Autodesk Inventor part; units mm, degrees
(part 2 of 2)
  spline S373 degree 2 poles (72.0686, 10.5759) (71.9893, 11.231) (71.9893, 11.5552) knots 0 0 0 1 1 1
  spline S374 degree 2 poles (76.8272, 9.9966) (76.7652, 9.9966) (76.541, 10.0724) (76.479, 10.0724) knots 0 0 0 1 2 2 2
  spline S375 degree 2 poles (76.479, 10.0724) (76.3548, 10.0724) (75.8514, 10.0414) (75.7203, 10.0414) knots 0 0 0 1 2 2 2
  spline S376 degree 2 poles (75.7203, 10.0414) (75.6238, 10.0414) (75.2479, 9.9931) (75.1514, 9.9931) knots 0 0 0 1 2 2 2
  spline S377 degree 2 poles (75.1514, 9.9931) (75.1238, 9.9931) (75.0203, 10.0138) (74.9927, 10.0138) knots 0 0 0 1 2 2 2
  spline S378 degree 2 poles (74.9927, 10.0138) (74.8238, 10.0138) (74.7721, 10.1793) knots 0 0 0 1 1 1
  spline S379 degree 2 poles (74.7721, 10.1793) (74.741, 10.2655) (74.741, 10.4759) knots 0 0 0 1 1 1
  spline S380 degree 2 poles (74.741, 10.4759) (74.741, 11.0517) (75.0548, 11.4034) knots 0 0 0 1 1 1
  spline S381 degree 2 poles (75.0548, 11.4034) (75.1996, 11.5621) (75.8272, 11.9966) knots 0 0 0 1 1 1
  spline S382 degree 2 poles (75.8272, 11.9966) (76.1824, 12.2379) (76.2996, 12.3759) knots 0 0 0 1 1 1
  spline S383 degree 2 poles (76.2996, 12.3759) (76.5134, 12.6103) (76.5134, 12.931) knots 0 0 0 1 1 1
  spline S384 degree 2 poles (76.5134, 12.931) (76.5134, 13.0897) (76.31, 13.2138) knots 0 0 0 1 1 1
  spline S385 degree 2 poles (76.31, 13.2138) (76.1272, 13.3241) (75.9548, 13.3241) knots 0 0 0 1 1 1
  spline S386 degree 2 poles (75.9548, 13.3241) (75.7272, 13.3241) (75.5238, 13.1931) knots 0 0 0 1 1 1
  line L70 (75.5238, 13.1931) -> (75.1686, 12.9138)
  spline S387 degree 2 poles (75.1686, 12.9138) (75.0617, 12.831) (74.9996, 12.831) knots 0 0 0 1 1 1
  spline S388 degree 2 poles (74.9996, 12.831) (74.7445, 12.831) (74.7445, 13.0345) knots 0 0 0 1 1 1
  spline S389 degree 2 poles (74.7445, 13.0345) (74.7445, 13.1517) (74.8376, 13.2345) knots 0 0 0 1 1 1
  spline S390 degree 2 poles (74.8376, 13.2345) (75.1272, 13.5069) (75.341, 13.6276) knots 0 0 0 1 1 1
  spline S391 degree 2 poles (75.341, 13.6276) (75.6376, 13.8) (75.9548, 13.8) knots 0 0 0 1 1 1
  spline S392 degree 2 poles (75.9548, 13.8) (76.3548, 13.8) (76.6686, 13.5828) knots 0 0 0 1 1 1
  spline S393 degree 2 poles (76.6686, 13.5828) (77.0203, 13.3379) (77.0203, 12.9552) knots 0 0 0 1 1 1
  spline S394 degree 2 poles (77.0203, 12.9552) (77.0203, 12.7) (76.8755, 12.2759) (76.7307, 12.1) knots 0 0 0 1 2 2 2
  spline S395 degree 2 poles (76.7307, 12.1) (76.5445, 11.8759) (76.1031, 11.6034) knots 0 0 0 1 1 1
  spline S396 degree 2 poles (76.1031, 11.6034) (75.6376, 11.3103) (75.4927, 11.1586) knots 0 0 0 1 1 1
  spline S397 degree 2 poles (75.4927, 11.1586) (75.2203, 10.8759) (75.2238, 10.469) knots 0 0 0 1 1 1
  line L71 (75.2238, 10.469) -> (75.7341, 10.5138)
  spline S398 degree 2 poles (75.7341, 10.5138) (76.2548, 10.5448) (76.479, 10.5448) knots 0 0 0 1 1 1
  spline S399 degree 2 poles (76.479, 10.5448) (76.6686, 10.5448) (76.8376, 10.4793) knots 0 0 0 1 1 1
  spline S400 degree 2 poles (76.8376, 10.4793) (77.0583, 10.3966) (77.0583, 10.2414) knots 0 0 0 1 1 1
  spline S401 degree 2 poles (77.0583, 10.2414) (77.0583, 10.1483) (76.9238, 9.9966) (76.8272, 9.9966) knots 0 0 0 1 2 2 2
  spline S402 degree 2 poles (80.279, 9.9) (79.9031, 9.9) (79.21, 10.5586) knots 0 0 0 1 1 1
  line L72 (79.21, 10.5586) -> (78.4686, 11.3034)
  line L73 (78.4686, 11.3034) -> (78.4686, 11.269)
  line L74 (78.4686, 11.269) -> (78.4686, 9.9724)
  spline S403 degree 2 poles (78.4686, 9.9724) (78.4686, 9.7276) (78.2548, 9.7276) knots 0 0 0 1 1 1
  spline S404 degree 2 poles (78.2548, 9.7276) (78.1134, 9.7276) (78.0272, 9.8517) knots 0 0 0 1 1 1
  spline S405 degree 2 poles (78.0272, 9.8517) (77.9583, 9.9517) (77.9583, 10.0724) knots 0 0 0 1 1 1
  spline S406 degree 2 poles (77.9583, 10.0724) (77.9583, 10.6517) (78.0272, 12.9552) (78.0272, 13.531) knots 0 0 0 1 2 2 2
  spline S407 degree 2 poles (78.0272, 13.531) (78.0272, 13.6379) (78.1686, 13.7862) (78.2721, 13.7862) knots 0 0 0 1 2 2 2
  spline S408 degree 2 poles (78.2721, 13.7862) (78.379, 13.7862) (78.5203, 13.6379) (78.5203, 13.531) knots 0 0 0 1 2 2 2
  spline S409 degree 2 poles (78.5203, 13.531) (78.5203, 13.2931) (78.4927, 12.7862) knots 0 0 0 1 1 1
  spline S410 degree 2 poles (78.4927, 12.7862) (78.4617, 12.2966) (78.4652, 12.0345) knots 0 0 0 1 1 1
  spline S411 degree 2 poles (78.4652, 12.0345) (78.7962, 12.3483) (79.2134, 12.8241) knots 0 0 0 1 1 1
  line L75 (79.2134, 12.8241) -> (79.9203, 13.6483)
  spline S412 degree 2 poles (79.9203, 13.6483) (80.0031, 13.7448) (80.11, 13.7448) knots 0 0 0 1 1 1
  spline S413 degree 2 poles (80.11, 13.7448) (80.2065, 13.7448) (80.3617, 13.5966) (80.3617, 13.4897) knots 0 0 0 1 2 2 2
  spline S414 degree 2 poles (80.3617, 13.4897) (80.3617, 13.3276) (79.7238, 12.6207) knots 0 0 0 1 1 1
  spline S415 degree 2 poles (79.7238, 12.6207) (79.2859, 12.1379) (78.8169, 11.6724) knots 0 0 0 1 1 1
  spline S416 degree 2 poles (78.8169, 11.6724) (79.1134, 11.3621) (79.7445, 10.7793) knots 0 0 0 1 1 1
  line L76 (79.7445, 10.7793) -> (80.0031, 10.5621)
  spline S417 degree 2 poles (80.0031, 10.5621) (80.1445, 10.4552) (80.3065, 10.4) knots 0 0 0 1 1 1
  spline S418 degree 2 poles (80.3065, 10.4) (80.5031, 10.3345) (80.5031, 10.1552) knots 0 0 0 1 1 1
  spline S419 degree 2 poles (80.5031, 10.1552) (80.5031, 10.069) (80.4514, 9.9931) knots 0 0 0 1 1 1
  spline S420 degree 2 poles (80.4514, 9.9931) (80.3859, 9.9) (80.279, 9.9) knots 0 0 0 1 1 1
  spline S421 degree 2 poles (83.0134, 9.9966) (82.9514, 9.9966) (82.7272, 10.0724) (82.6652, 10.0724) knots 0 0 0 1 2 2 2
  spline S422 degree 2 poles (82.6652, 10.0724) (82.541, 10.0724) (82.0376, 10.0414) (81.9065, 10.0414) knots 0 0 0 1 2 2 2
  spline S423 degree 2 poles (81.9065, 10.0414) (81.81, 10.0414) (81.4341, 9.9931) (81.3376, 9.9931) knots 0 0 0 1 2 2 2
  spline S424 degree 2 poles (81.3376, 9.9931) (81.31, 9.9931) (81.2065, 10.0138) (81.179, 10.0138) knots 0 0 0 1 2 2 2
  spline S425 degree 2 poles (81.179, 10.0138) (81.01, 10.0138) (80.9583, 10.1793) knots 0 0 0 1 1 1
  spline S426 degree 2 poles (80.9583, 10.1793) (80.9272, 10.2655) (80.9272, 10.4759) knots 0 0 0 1 1 1
  spline S427 degree 2 poles (80.9272, 10.4759) (80.9272, 11.0517) (81.241, 11.4034) knots 0 0 0 1 1 1
  spline S428 degree 2 poles (81.241, 11.4034) (81.3859, 11.5621) (82.0134, 11.9966) knots 0 0 0 1 1 1
  spline S429 degree 2 poles (82.0134, 11.9966) (82.3686, 12.2379) (82.4859, 12.3759) knots 0 0 0 1 1 1
  spline S430 degree 2 poles (82.4859, 12.3759) (82.6996, 12.6103) (82.6996, 12.931) knots 0 0 0 1 1 1
  spline S431 degree 2 poles (82.6996, 12.931) (82.6996, 13.0897) (82.4962, 13.2138) knots 0 0 0 1 1 1
  spline S432 degree 2 poles (82.4962, 13.2138) (82.3134, 13.3241) (82.141, 13.3241) knots 0 0 0 1 1 1
  spline S433 degree 2 poles (82.141, 13.3241) (81.9134, 13.3241) (81.71, 13.1931) knots 0 0 0 1 1 1
  line L77 (81.71, 13.1931) -> (81.3548, 12.9138)
  spline S434 degree 2 poles (81.3548, 12.9138) (81.2479, 12.831) (81.1859, 12.831) knots 0 0 0 1 1 1
  spline S435 degree 2 poles (81.1859, 12.831) (80.9307, 12.831) (80.9307, 13.0345) knots 0 0 0 1 1 1
  spline S436 degree 2 poles (80.9307, 13.0345) (80.9307, 13.1517) (81.0238, 13.2345) knots 0 0 0 1 1 1
  spline S437 degree 2 poles (81.0238, 13.2345) (81.3134, 13.5069) (81.5272, 13.6276) knots 0 0 0 1 1 1
  spline S438 degree 2 poles (81.5272, 13.6276) (81.8238, 13.8) (82.141, 13.8) knots 0 0 0 1 1 1
  spline S439 degree 2 poles (82.141, 13.8) (82.541, 13.8) (82.8548, 13.5828) knots 0 0 0 1 1 1
  spline S440 degree 2 poles (82.8548, 13.5828) (83.2065, 13.3379) (83.2065, 12.9552) knots 0 0 0 1 1 1
  spline S441 degree 2 poles (83.2065, 12.9552) (83.2065, 12.7) (83.0617, 12.2759) (82.9169, 12.1) knots 0 0 0 1 2 2 2
  spline S442 degree 2 poles (82.9169, 12.1) (82.7307, 11.8759) (82.2893, 11.6034) knots 0 0 0 1 1 1
  spline S443 degree 2 poles (82.2893, 11.6034) (81.8238, 11.3103) (81.679, 11.1586) knots 0 0 0 1 1 1
  spline S444 degree 2 poles (81.679, 11.1586) (81.4065, 10.8759) (81.41, 10.469) knots 0 0 0 1 1 1
  line L78 (81.41, 10.469) -> (81.9203, 10.5138)
  spline S445 degree 2 poles (81.9203, 10.5138) (82.441, 10.5448) (82.6652, 10.5448) knots 0 0 0 1 1 1
  spline S446 degree 2 poles (82.6652, 10.5448) (82.8548, 10.5448) (83.0238, 10.4793) knots 0 0 0 1 1 1
  spline S447 degree 2 poles (83.0238, 10.4793) (83.2445, 10.3966) (83.2445, 10.2414) knots 0 0 0 1 1 1
  spline S448 degree 2 poles (83.2445, 10.2414) (83.2445, 10.1483) (83.11, 9.9966) (83.0134, 9.9966) knots 0 0 0 1 2 2 2
  spline S449 degree 2 poles (85.0927, 9.8207) (84.4445, 9.8207) (84.141, 10.2931) knots 0 0 0 1 1 1
  spline S450 degree 2 poles (84.141, 10.2931) (83.8893, 10.6828) (83.8893, 11.331) knots 0 0 0 1 1 1
  spline S451 degree 2 poles (83.8893, 11.331) (83.8893, 12.5517) (84.8824, 13.4483) knots 0 0 0 1 1 1
  line L79 (84.8824, 13.4483) -> (85.1134, 13.6862)
  spline S452 degree 2 poles (85.1134, 13.6862) (85.2824, 13.8483) (85.3721, 13.8483) knots 0 0 0 1 1 1
  spline S453 degree 2 poles (85.3721, 13.8483) (85.4686, 13.8483) (85.6169, 13.7069) (85.6203, 13.6103) knots 0 0 0 1 2 2 2
  spline S454 degree 2 poles (85.6203, 13.6103) (85.6238, 13.5207) (85.3686, 13.269) knots 0 0 0 1 1 1
  line L80 (85.3686, 13.269) -> (84.8617, 12.7759)
  spline S455 degree 2 poles (84.8617, 12.7759) (84.6617, 12.5724) (84.5203, 12.1621) knots 0 0 0 1 1 1
  spline S456 degree 2 poles (84.5203, 12.1621) (84.7341, 12.2621) (85.0548, 12.3586) (85.1617, 12.3586) knots 0 0 0 1 2 2 2
  spline S457 degree 2 poles (85.1617, 12.3586) (85.741, 12.3586) (86.3583, 11.7379) (86.3583, 11.1759) knots 0 0 0 1 2 2 2
  spline S458 degree 2 poles (86.3583, 11.1759) (86.3583, 10.5828) (86.0238, 10.2103) knots 0 0 0 1 1 1
  spline S459 degree 2 poles (86.0238, 10.2103) (85.6755, 9.8207) (85.0927, 9.8207) knots 0 0 0 1 1 1
  spline S460 degree 2 poles (85.0927, 11.8552) (84.879, 11.8552) (84.71, 11.7793) knots 0 0 0 1 1 1
  spline S461 degree 2 poles (84.71, 11.7793) (84.6445, 11.7517) (84.3859, 11.5897) knots 0 0 0 1 1 1
  spline S462 degree 2 poles (84.3859, 11.5897) (84.3721, 11.4586) (84.3721, 11.331) knots 0 0 0 1 1 1
  spline S463 degree 2 poles (84.3721, 11.331) (84.3721, 10.8897) (84.5203, 10.6103) knots 0 0 0 1 1 1
  spline S464 degree 2 poles (84.5203, 10.6103) (84.71, 10.2517) (85.1065, 10.2517) knots 0 0 0 1 1 1
  spline S465 degree 2 poles (85.1065, 10.2517) (85.479, 10.2517) (85.6859, 10.5207) knots 0 0 0 1 1 1
  spline S466 degree 2 poles (85.6859, 10.5207) (85.8755, 10.7655) (85.8755, 11.1759) knots 0 0 0 1 1 1
  spline S467 degree 2 poles (85.8755, 11.1759) (85.8755, 11.5172) (85.4859, 11.8552) (85.0927, 11.8552) knots 0 0 0 1 2 2 2
  line L81 (4.6538, 4.8079) -> (3.1401, 4.8079)
  line L82 (3.1401, 4.8079) -> (3.1401, 5.2941)
  line L83 (3.1401, 5.2941) -> (4.6538, 5.2941)
  line L84 (4.6538, 5.2941) -> (4.6538, 4.8079)
  spline S468 degree 2 poles (8.132, 3.2292) (7.6976, 3.2292) (7.0882, 3.4108) (6.8191, 3.5404) knots 0 0 0 1 2 2 2
  line L85 (6.8191, 3.5404) -> (6.8191, 4.2082)
  line L86 (6.8191, 4.2082) -> (6.858, 4.2082)
  spline S469 degree 2 poles (6.858, 4.2082) (7.1206, 3.9618) (7.7851, 3.6895) (8.0931, 3.6895) knots 0 0 0 1 2 2 2
  spline S470 degree 2 poles (8.0931, 3.6895) (8.5339, 3.6895) (8.9845, 4.0558) (8.9845, 4.3573) knots 0 0 0 1 2 2 2
  spline S471 degree 2 poles (8.9845, 4.3573) (8.9845, 4.5972) (8.7478, 4.8954) (8.4918, 4.9699) knots 0 0 0 1 2 2 2
  spline S472 degree 2 poles (8.4918, 4.9699) (8.307, 5.0218) (7.9991, 5.0931) (7.7689, 5.1515) knots 0 0 0 1 2 2 2
  spline S473 degree 2 poles (7.7689, 5.1515) (7.5614, 5.2066) (7.2341, 5.3719) (7.1076, 5.5048) knots 0 0 0 1 2 2 2
  spline S474 degree 2 poles (7.1076, 5.5048) (6.9845, 5.6377) (6.8483, 5.9942) (6.8483, 6.2276) knots 0 0 0 1 2 2 2
  spline S475 degree 2 poles (6.8483, 6.2276) (6.8483, 6.7138) (7.6068, 7.3719) (8.1935, 7.3719) knots 0 0 0 1 2 2 2
  spline S476 degree 2 poles (8.1935, 7.3719) (8.5307, 7.3719) (9.1271, 7.239) (9.3832, 7.1126) knots 0 0 0 1 2 2 2
  line L87 (9.3832, 7.1126) -> (9.3832, 6.4772)
  line L88 (9.3832, 6.4772) -> (9.3443, 6.4772)
  spline S477 degree 2 poles (9.3443, 6.4772) (9.153, 6.6523) (8.5566, 6.9116) (8.2292, 6.9116) knots 0 0 0 1 2 2 2
  spline S478 degree 2 poles (8.2292, 6.9116) (7.8597, 6.9116) (7.4026, 6.5647) (7.4026, 6.2827) knots 0 0 0 1 2 2 2
  spline S479 degree 2 poles (7.4026, 6.2827) (7.4026, 6.0299) (7.6717, 5.7284) (7.9245, 5.6604) knots 0 0 0 1 2 2 2
  spline S480 degree 2 poles (7.9245, 5.6604) (8.0931, 5.615) (8.5825, 5.4983) (8.7446, 5.4497) knots 0 0 0 1 2 2 2
  spline S481 degree 2 poles (8.7446, 5.4497) (9.1563, 5.3232) (9.5388, 4.8143) (9.5388, 4.4416) knots 0 0 0 1 2 2 2
  spline S482 degree 2 poles (9.5388, 4.4416) (9.5388, 4.2049) (9.3475, 3.7511) (9.1757, 3.5923) knots 0 0 0 1 2 2 2
  spline S483 degree 2 poles (9.1757, 3.5923) (8.9845, 3.4173) (8.4982, 3.2292) (8.132, 3.2292) knots 0 0 0 1 2 2 2
  spline S484 degree 2 poles (12.508, 4.8014) (12.508, 4.0429) (11.7786, 3.2163) (11.1692, 3.2163) knots 0 0 0 1 2 2 2
  spline S485 degree 2 poles (11.1692, 3.2163) (10.5436, 3.2163) (9.8273, 4.0688) (9.8273, 4.8014) knots 0 0 0 1 2 2 2
  spline S486 degree 2 poles (9.8273, 4.8014) (9.8273, 5.5534) (10.5663, 6.3865) (11.1692, 6.3865) knots 0 0 0 1 2 2 2
  spline S487 degree 2 poles (11.1692, 6.3865) (11.7786, 6.3865) (12.508, 5.5566) (12.508, 4.8014) knots 0 0 0 1 2 2 2
  spline S488 degree 2 poles (11.9861, 4.8014) (11.9861, 5.3848) (11.5614, 5.9521) (11.1692, 5.9521) knots 0 0 0 1 2 2 2
  spline S489 degree 2 poles (11.1692, 5.9521) (10.777, 5.9521) (10.3491, 5.3848) (10.3491, 4.8014) knots 0 0 0 1 2 2 2
  spline S490 degree 2 poles (10.3491, 4.8014) (10.3491, 4.2341) (10.777, 3.6506) (11.1692, 3.6506) knots 0 0 0 1 2 2 2
  spline S491 degree 2 poles (11.1692, 3.6506) (11.5582, 3.6506) (11.9861, 4.2244) (11.9861, 4.8014) knots 0 0 0 1 2 2 2
  spline S492 degree 2 poles (15.4934, 4.8014) (15.4934, 4.0429) (14.764, 3.2163) (14.1546, 3.2163) knots 0 0 0 1 2 2 2
  spline S493 degree 2 poles (14.1546, 3.2163) (13.529, 3.2163) (12.8127, 4.0688) (12.8127, 4.8014) knots 0 0 0 1 2 2 2
  spline S494 degree 2 poles (12.8127, 4.8014) (12.8127, 5.5534) (13.5517, 6.3865) (14.1546, 6.3865) knots 0 0 0 1 2 2 2
  spline S495 degree 2 poles (14.1546, 6.3865) (14.764, 6.3865) (15.4934, 5.5566) (15.4934, 4.8014) knots 0 0 0 1 2 2 2
  spline S496 degree 2 poles (14.9715, 4.8014) (14.9715, 5.3848) (14.5469, 5.9521) (14.1546, 5.9521) knots 0 0 0 1 2 2 2
  spline S497 degree 2 poles (14.1546, 5.9521) (13.7624, 5.9521) (13.3345, 5.3848) (13.3345, 4.8014) knots 0 0 0 1 2 2 2
  spline S498 degree 2 poles (13.3345, 4.8014) (13.3345, 4.2341) (13.7624, 3.6506) (14.1546, 3.6506) knots 0 0 0 1 2 2 2
  spline S499 degree 2 poles (14.1546, 3.6506) (14.5436, 3.6506) (14.9715, 4.2244) (14.9715, 4.8014) knots 0 0 0 1 2 2 2
  line L89 (18.3686, 3.3006) -> (16.0509, 3.3006)
  line L90 (16.0509, 3.3006) -> (16.0509, 7.3006)
  line L91 (16.0509, 7.3006) -> (16.5825, 7.3006)
  line L92 (16.5825, 7.3006) -> (16.5825, 3.7738)
  line L93 (16.5825, 3.7738) -> (18.3686, 3.7738)
  line L94 (18.3686, 3.7738) -> (18.3686, 3.3006)
  spline S500 degree 2 poles (20.4204, 3.6182) (20.3589, 3.5728) (20.1514, 3.4108) (20.0542, 3.3621) knots 0 0 0 1 2 2 2
  spline S501 degree 2 poles (20.0542, 3.3621) (19.9213, 3.2908) (19.6717, 3.2163) (19.4448, 3.2163) knots 0 0 0 1 2 2 2
  spline S502 degree 2 poles (19.4448, 3.2163) (19.26, 3.2163) (18.9261, 3.3557) (18.7997, 3.4821) knots 0 0 0 1 2 2 2
  spline S503 degree 2 poles (18.7997, 3.4821) (18.6798, 3.6053) (18.5339, 3.9683) (18.5339, 4.1693) knots 0 0 0 1 2 2 2
  spline S504 degree 2 poles (18.5339, 4.1693) (18.5339, 4.4805) (18.7965, 4.9213) (19.0817, 5.0477) knots 0 0 0 1 2 2 2
  spline S505 degree 2 poles (19.0817, 5.0477) (19.3345, 5.1644) (20.0217, 5.2519) (20.4204, 5.2746) knots 0 0 0 1 2 2 2
  line L95 (20.4204, 5.2746) -> (20.4204, 5.3719)
  spline S506 degree 2 poles (20.4204, 5.3719) (20.4204, 5.5469) (20.3135, 5.7641) (20.2162, 5.8257) knots 0 0 0 1 2 2 2
  spline S507 degree 2 poles (20.2162, 5.8257) (20.119, 5.8873) (19.8402, 5.9262) (19.6911, 5.9262) knots 0 0 0 1 2 2 2
  spline S508 degree 2 poles (19.6911, 5.9262) (19.5161, 5.9262) (19.0428, 5.8224) (18.8062, 5.722) knots 0 0 0 1 2 2 2
  line L96 (18.8062, 5.722) -> (18.777, 5.722)
  line L97 (18.777, 5.722) -> (18.777, 6.2374)
  spline S509 degree 2 poles (18.777, 6.2374) (18.9164, 6.2762) (19.4383, 6.3735) (19.6944, 6.3735) knots 0 0 0 1 2 2 2
  spline S510 degree 2 poles (19.6944, 6.3735) (20.0055, 6.3735) (20.4302, 6.2762) (20.5987, 6.1498) knots 0 0 0 1 2 2 2
  spline S511 degree 2 poles (20.5987, 6.1498) (20.764, 6.0267) (20.9261, 5.6344) (20.9261, 5.3524) knots 0 0 0 1 2 2 2
  line L98 (20.9261, 5.3524) -> (20.9261, 3.3006)
  line L99 (20.9261, 3.3006) -> (20.4204, 3.3006)
  line L100 (20.4204, 3.3006) -> (20.4204, 3.6182)
  line L101 (20.4204, 4.0396) -> (20.4204, 4.8727)
  spline S512 degree 2 poles (20.4204, 4.8727) (20.2389, 4.8565) (19.6911, 4.8014) (19.5193, 4.7495) knots 0 0 0 1 2 2 2
  spline S513 degree 2 poles (19.5193, 4.7495) (19.3183, 4.6879) (19.0558, 4.4318) (19.0558, 4.2049) knots 0 0 0 1 2 2 2
  spline S514 degree 2 poles (19.0558, 4.2049) (19.0558, 3.9456) (19.3475, 3.6831) (19.6263, 3.6831) knots 0 0 0 1 2 2 2
  spline S515 degree 2 poles (19.6263, 3.6831) (19.8629, 3.6831) (20.2519, 3.8873) (20.4204, 4.0396) knots 0 0 0 1 2 2 2
  spline S516 degree 2 poles (24.1514, 4.85) (24.1514, 4.1142) (23.4383, 3.2163) (22.9002, 3.2163) knots 0 0 0 1 2 2 2
  spline S517 degree 2 poles (22.9002, 3.2163) (22.6571, 3.2163) (22.3102, 3.3362) (22.1417, 3.4399) knots 0 0 0 1 2 2 2
  line L102 (22.1417, 3.4399) -> (22.1093, 3.3006)
  line L103 (22.1093, 3.3006) -> (21.636, 3.3006)
  line L104 (21.636, 3.3006) -> (21.636, 7.4788)
  line L105 (21.636, 7.4788) -> (22.1417, 7.4788)
  line L106 (22.1417, 7.4788) -> (22.1417, 5.9878)
  spline S518 degree 2 poles (22.1417, 5.9878) (22.3329, 6.1596) (22.777, 6.3865) (23.059, 6.3865) knots 0 0 0 1 2 2 2
  spline S519 degree 2 poles (23.059, 6.3865) (23.5679, 6.3865) (24.1514, 5.5728) (24.1514, 4.85) knots 0 0 0 1 2 2 2
  spline S520 degree 2 poles (23.6295, 4.8111) (23.6295, 5.3492) (23.3021, 5.9067) (22.9391, 5.9067) knots 0 0 0 1 2 2 2
  spline S521 degree 2 poles (22.9391, 5.9067) (22.7349, 5.9067) (22.3135, 5.7122) (22.1417, 5.5631) knots 0 0 0 1 2 2 2
  line L107 (22.1417, 5.5631) -> (22.1417, 3.8419)
  spline S522 degree 2 poles (22.1417, 3.8419) (22.3329, 3.7479) (22.6279, 3.6701) (22.8029, 3.6701) knots 0 0 0 1 2 2 2
  spline S523 degree 2 poles (22.8029, 3.6701) (23.1887, 3.6701) (23.6295, 4.2179) (23.6295, 4.8111) knots 0 0 0 1 2 2 2
  line L108 (74.1709, 4.8079) -> (72.6571, 4.8079)
  line L109 (72.6571, 4.8079) -> (72.6571, 5.2941)
  line L110 (72.6571, 5.2941) -> (74.1709, 5.2941)
  line L111 (74.1709, 5.2941) -> (74.1709, 4.8079)
  line L112 (77.8726, 4.8889) -> (74.9877, 3.5113)
  line L113 (74.9877, 3.5113) -> (74.9877, 3.9878)
  line L114 (74.9877, 3.9878) -> (77.2243, 5.051)
  line L115 (77.2243, 5.051) -> (74.9877, 6.1109)
  line L116 (74.9877, 6.1109) -> (74.9877, 6.5874)
  line L117 (74.9877, 6.5874) -> (77.8726, 5.2098)
  line L118 (77.8726, 5.2098) -> (77.8726, 4.8889)
  line L119 (83.9666, 3.3006) -> (83.435, 3.3006)
  line L120 (83.435, 3.3006) -> (83.435, 6.7463)
  line L121 (83.435, 6.7463) -> (82.3913, 4.4027)
  line L122 (82.3913, 4.4027) -> (82.0671, 4.4027)
  line L123 (82.0671, 4.4027) -> (81.0331, 6.7463)
  line L124 (81.0331, 6.7463) -> (81.0331, 3.3006)
  line L125 (81.0331, 3.3006) -> (80.5371, 3.3006)
  line L126 (80.5371, 3.3006) -> (80.5371, 7.3006)
  line L127 (80.5371, 7.3006) -> (81.2632, 7.3006)
  line L128 (81.2632, 7.3006) -> (82.2616, 5.0737)
  line L129 (82.2616, 5.0737) -> (83.2276, 7.3006)
  line L130 (83.2276, 7.3006) -> (83.9666, 7.3006)
  line L131 (83.9666, 7.3006) -> (83.9666, 3.3006)
  spline S524 degree 2 poles (86.4107, 3.6182) (86.3491, 3.5728) (86.1417, 3.4108) (86.0444, 3.3621) knots 0 0 0 1 2 2 2
  spline S525 degree 2 poles (86.0444, 3.3621) (85.9115, 3.2908) (85.6619, 3.2163) (85.435, 3.2163) knots 0 0 0 1 2 2 2
  spline S526 degree 2 poles (85.435, 3.2163) (85.2503, 3.2163) (84.9164, 3.3557) (84.79, 3.4821) knots 0 0 0 1 2 2 2
  spline S527 degree 2 poles (84.79, 3.4821) (84.67, 3.6053) (84.5242, 3.9683) (84.5242, 4.1693) knots 0 0 0 1 2 2 2
  spline S528 degree 2 poles (84.5242, 4.1693) (84.5242, 4.4805) (84.7867, 4.9213) (85.072, 5.0477) knots 0 0 0 1 2 2 2
  spline S529 degree 2 poles (85.072, 5.0477) (85.3248, 5.1644) (86.012, 5.2519) (86.4107, 5.2746) knots 0 0 0 1 2 2 2
  line L132 (86.4107, 5.2746) -> (86.4107, 5.3719)
  spline S530 degree 2 poles (86.4107, 5.3719) (86.4107, 5.5469) (86.3038, 5.7641) (86.2065, 5.8257) knots 0 0 0 1 2 2 2
  spline S531 degree 2 poles (86.2065, 5.8257) (86.1093, 5.8873) (85.8305, 5.9262) (85.6814, 5.9262) knots 0 0 0 1 2 2 2
  spline S532 degree 2 poles (85.6814, 5.9262) (85.5063, 5.9262) (85.0331, 5.8224) (84.7965, 5.722) knots 0 0 0 1 2 2 2
  line L133 (84.7965, 5.722) -> (84.7673, 5.722)
  line L134 (84.7673, 5.722) -> (84.7673, 6.2374)
  spline S533 degree 2 poles (84.7673, 6.2374) (84.9067, 6.2762) (85.4286, 6.3735) (85.6846, 6.3735) knots 0 0 0 1 2 2 2
  spline S534 degree 2 poles (85.6846, 6.3735) (85.9958, 6.3735) (86.4204, 6.2762) (86.589, 6.1498) knots 0 0 0 1 2 2 2
  spline S535 degree 2 poles (86.589, 6.1498) (86.7543, 6.0267) (86.9164, 5.6344) (86.9164, 5.3524) knots 0 0 0 1 2 2 2
  line L135 (86.9164, 5.3524) -> (86.9164, 3.3006)
  line L136 (86.9164, 3.3006) -> (86.4107, 3.3006)
  line L137 (86.4107, 3.3006) -> (86.4107, 3.6182)
  line L138 (86.4107, 4.0396) -> (86.4107, 4.8727)
  spline S536 degree 2 poles (86.4107, 4.8727) (86.2292, 4.8565) (85.6814, 4.8014) (85.5096, 4.7495) knots 0 0 0 1 2 2 2
  spline S537 degree 2 poles (85.5096, 4.7495) (85.3086, 4.6879) (85.0461, 4.4318) (85.0461, 4.2049) knots 0 0 0 1 2 2 2
  spline S538 degree 2 poles (85.0461, 4.2049) (85.0461, 3.9456) (85.3378, 3.6831) (85.6166, 3.6831) knots 0 0 0 1 2 2 2
  spline S539 degree 2 poles (85.6166, 3.6831) (85.8532, 3.6831) (86.2422, 3.8873) (86.4107, 4.0396) knots 0 0 0 1 2 2 2
  spline S540 degree 2 poles (88.5339, 3.2422) (88.1222, 3.2422) (87.6587, 3.7122) (87.6587, 4.2211) knots 0 0 0 1 2 2 2
  line L139 (87.6587, 4.2211) -> (87.6587, 5.884)
  line L140 (87.6587, 5.884) -> (87.3183, 5.884)
  line L141 (87.3183, 5.884) -> (87.3183, 6.3022)
  line L142 (87.3183, 6.3022) -> (87.6587, 6.3022)
  line L143 (87.6587, 6.3022) -> (87.6587, 7.1644)
  line L144 (87.6587, 7.1644) -> (88.1644, 7.1644)
  line L145 (88.1644, 7.1644) -> (88.1644, 6.3022)
  line L146 (88.1644, 6.3022) -> (89.0947, 6.3022)
  line L147 (89.0947, 6.3022) -> (89.0947, 5.884)
  line L148 (89.0947, 5.884) -> (88.1644, 5.884)
  line L149 (88.1644, 5.884) -> (88.1644, 4.4545)
  spline S541 degree 2 poles (88.1644, 4.4545) (88.1644, 4.2276) (88.1806, 3.978) (88.2357, 3.8711) knots 0 0 0 1 2 2 2
  spline S542 degree 2 poles (88.2357, 3.8711) (88.2811, 3.7771) (88.4853, 3.6831) (88.6603, 3.6831) knots 0 0 0 1 2 2 2
  spline S543 degree 2 poles (88.6603, 3.6831) (88.7835, 3.6831) (89.0136, 3.7576) (89.0655, 3.7803) knots 0 0 0 1 2 2 2
  line L150 (89.0655, 3.7803) -> (89.0947, 3.7803)
  line L151 (89.0947, 3.7803) -> (89.0947, 3.3265)
  spline S544 degree 2 poles (89.0947, 3.3265) (88.9521, 3.2876) (88.6603, 3.2422) (88.5339, 3.2422) knots 0 0 0 1 2 2 2
  spline S545 degree 2 poles (90.7705, 3.2325) (90.0509, 3.2325) (89.26, 4.0396) (89.26, 4.7852) knots 0 0 0 1 2 2 2
  spline S546 degree 2 poles (89.26, 4.7852) (89.26, 5.5177) (90.0282, 6.3865) (90.6474, 6.3865) knots 0 0 0 1 2 2 2
  spline S547 degree 2 poles (90.6474, 6.3865) (90.9261, 6.3865) (91.3572, 6.2244) (91.5161, 6.0526) knots 0 0 0 1 2 2 2
  spline S548 degree 2 poles (91.5161, 6.0526) (91.6781, 5.8808) (91.8499, 5.3848) (91.8499, 5.025) knots 0 0 0 1 2 2 2
  line L152 (91.8499, 5.025) -> (91.8499, 4.7495)
  line L153 (91.8499, 4.7495) -> (89.7721, 4.7495)
  spline S549 degree 2 poles (89.7721, 4.7495) (89.7721, 4.2276) (90.2973, 3.6733) (90.764, 3.6733) knots 0 0 0 1 2 2 2
  spline S550 degree 2 poles (90.764, 3.6733) (90.9294, 3.6733) (91.2503, 3.7479) (91.3799, 3.8062) knots 0 0 0 1 2 2 2
  spline S551 degree 2 poles (91.3799, 3.8062) (91.5161, 3.8711) (91.7041, 3.9845) (91.7657, 4.0364) knots 0 0 0 1 2 2 2
  line L154 (91.7657, 4.0364) -> (91.7948, 4.0364)
  line L155 (91.7948, 4.0364) -> (91.7948, 3.4853)
  spline S552 degree 2 poles (91.7948, 3.4853) (91.7073, 3.4497) (91.4415, 3.3459) (91.3378, 3.3168) knots 0 0 0 1 2 2 2
  spline S553 degree 2 poles (91.3378, 3.3168) (91.1919, 3.2746) (90.9521, 3.2325) (90.7705, 3.2325) knots 0 0 0 1 2 2 2
  spline S554 degree 2 poles (91.3572, 5.1352) (91.3508, 5.3395) (91.2665, 5.6377) (91.1854, 5.7382) knots 0 0 0 1 2 2 2
  spline S555 degree 2 poles (91.1854, 5.7382) (91.0979, 5.8516) (90.8224, 5.9715) (90.6182, 5.9715) knots 0 0 0 1 2 2 2
  spline S556 degree 2 poles (90.6182, 5.9715) (90.4172, 5.9715) (90.1352, 5.8516) (90.0185, 5.7349) knots 0 0 0 1 2 2 2
  spline S557 degree 2 poles (90.0185, 5.7349) (89.905, 5.615) (89.7884, 5.3265) (89.7721, 5.1352) knots 0 0 0 1 2 2 2
  line L156 (89.7721, 5.1352) -> (91.3572, 5.1352)
  point P0 (48, -2)
  dimension "d41" = 10
  constraints: 2 end point, 2 horizontal, 2 point on circle
  measures "d41" distance between parallel lines of L1 L0
extrude "Extrusion10" cut sketch "Sketch12" against normal blind 1
body "Solid1"
